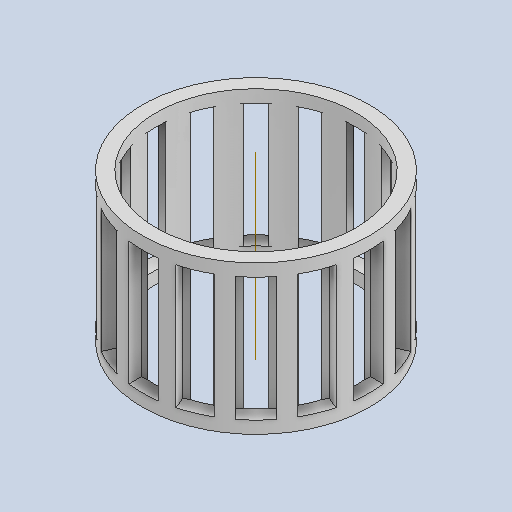
# Autodesk Inventor part: magnet_ring
Saved by Autodesk Inventor 2025 (Build 290162000, 162)
## iProperties
Created: 2026-08-03
Part Number: magnet_ring
Material: Ogólny
Document SubType Name: Modeling
Designer: zzapa
Density: 1 g/cm^3
Appearance: Domyślna
Author: zzapa
Autodesk Inventor part; units mm, degrees
ref_plane "YZ Plane" through (0, 0, 0) normal (1, 0, 0) x (0, 1, 0)
ref_plane "XZ Plane" through (0, 0, 0) normal (0, 1, 0) x (-1, 0, 0)
ref_plane "XY Plane" through (0, 0, 0) normal (0, 0, 1) x (1, 0, 0)
sketch "Szkic1" plane through (0, 0, 0) normal (0, 0, 1) x (1, 0, 0)
  line L0 (27.5, 18) -> (24.2, 18)
  line L1 (24.2, 18) -> (24.2, -18)
  line L2 (24.2, -18) -> (27.5, -18)
  line L3 (27.5, -18) -> (27.5, 18)
  line L4 (-5.5, 0) -> (33, 0) projected
  line L5 (0, -25.2) -> (0, 25.2) projected
  point P0 (0, 0)
  point P1 (24.2, 0)
  dimension "d0" = 27.5
  dimension "d1" = 3.3
  dimension "d15" = 36
  constraints: 8 end point, 2 parallel, 1 horizontal, 1 midpoint, 1 perpendicular, 1 point on line
  measures "d0" distance from line of point (0, 0) L3
  measures "d1" distance of L0.start L0.end
  measures "d15" distance of L2.end L0.start
revolve "Obrót1" add sketch "Szkic1" angle 360 about axis through (0, -10, 0) along (0, 1, 0)
sketch "Szkic2" plane through (0, 0, 0) normal (0, 1, 0) x (-1, 0, 0)
  line L0 (24.1699, -3.55) -> (27.2699, -3.55)
  line L1 (27.2699, -3.55) -> (27.2699, 3.55)
  line L2 (27.2699, 3.55) -> (24.1699, 3.55)
  line L3 (24.1699, 3.55) -> (24.1699, -3.55)
  circle A0 centre (0, 0) radius 27.5 projected
  line L4 (38.5, 0) -> (-38.5, 0) projected
  line L5 (27.2699, -3.55) -> (27.5, -3.55)
  line L6 (27.5, -3.55) -> (27.5, 3.55)
  line L7 (27.5, 3.55) -> (27.2699, 3.55)
  line L8 (27.2699, 3.55) -> (27.2699, -3.55)
  line L9 (24.1043, -2.15) -> (24.1699, -2.15)
  line L10 (24.1699, -2.15) -> (24.1699, 2.15)
  line L11 (24.1699, 2.15) -> (24.1043, 2.15)
  line L12 (24.1043, 2.15) -> (24.1043, -2.15)
  circle A1 centre (0, 0) radius 24.2 projected
  line L13 (23.0922, 7.238) -> (23.1528, 7.2631)
  line L14 (21.4467, 11.2107) -> (23.0922, 7.238)
  line L15 (23.1528, 7.2631) -> (21.5073, 11.2358)
  line L16 (20.9716, 12.5292) -> (23.6886, 5.9696)
  line L17 (23.6886, 5.9696) -> (26.5526, 7.156)
  line L18 (23.8356, 13.7155) -> (20.9716, 12.5292)
  line L19 (26.5526, 7.156) -> (26.7652, 7.244)
  line L20 (24.0482, 13.8036) -> (23.8356, 13.7155)
  line L21 (26.5526, 7.156) -> (23.8356, 13.7155)
  line L22 (23.8356, 13.7155) -> (26.5526, 7.156)
  line L23 (26.7652, 7.244) -> (24.0482, 13.8036)
  line L24 (21.5073, 11.2358) -> (21.4467, 11.2107)
  line L25 (18.5646, 15.524) -> (18.611, 15.5704)
  line L26 (15.524, 18.5646) -> (18.5646, 15.524)
  line L27 (18.611, 15.5704) -> (15.5704, 18.611)
  line L28 (14.5805, 19.6009) -> (19.6009, 14.5805)
  line L29 (19.6009, 14.5805) -> (21.793, 16.7725)
  line L30 (16.7725, 21.793) -> (14.5805, 19.6009)
  line L31 (21.793, 16.7725) -> (21.9557, 16.9352)
  line L32 (16.9352, 21.9557) -> (16.7725, 21.793)
  line L33 (21.793, 16.7725) -> (16.7725, 21.793)
  line L34 (16.7725, 21.793) -> (21.793, 16.7725)
  line L35 (21.9557, 16.9352) -> (16.9352, 21.9557)
  line L36 (15.5704, 18.611) -> (15.524, 18.5646)
  line L37 (11.2107, 21.4467) -> (11.2358, 21.5073)
  line L38 (7.238, 23.0922) -> (11.2107, 21.4467)
  line L39 (11.2358, 21.5073) -> (7.2631, 23.1528)
  line L40 (5.9696, 23.6886) -> (12.5292, 20.9716)
  line L41 (12.5292, 20.9716) -> (13.7155, 23.8356)
  line L42 (7.156, 26.5526) -> (5.9696, 23.6886)
  line L43 (13.7155, 23.8356) -> (13.8036, 24.0482)
  line L44 (7.244, 26.7652) -> (7.156, 26.5526)
  line L45 (13.7155, 23.8356) -> (7.156, 26.5526)
  line L46 (7.156, 26.5526) -> (13.7155, 23.8356)
  line L47 (13.8036, 24.0482) -> (7.244, 26.7652)
  line L48 (7.2631, 23.1528) -> (7.238, 23.0922)
  line L49 (2.15, 24.1043) -> (2.15, 24.1699)
  line L50 (-2.15, 24.1043) -> (2.15, 24.1043)
  line L51 (2.15, 24.1699) -> (-2.15, 24.1699)
  line L52 (-3.55, 24.1699) -> (3.55, 24.1699)
  line L53 (3.55, 24.1699) -> (3.55, 27.2699)
  line L54 (-3.55, 27.2699) -> (-3.55, 24.1699)
  line L55 (3.55, 27.2699) -> (3.55, 27.5)
  line L56 (-3.55, 27.5) -> (-3.55, 27.2699)
  line L57 (3.55, 27.2699) -> (-3.55, 27.2699)
  line L58 (-3.55, 27.2699) -> (3.55, 27.2699)
  line L59 (3.55, 27.5) -> (-3.55, 27.5)
  line L60 (-2.15, 24.1699) -> (-2.15, 24.1043)
  line L61 (-7.238, 23.0922) -> (-7.2631, 23.1528)
  line L62 (-11.2107, 21.4467) -> (-7.238, 23.0922)
  line L63 (-7.2631, 23.1528) -> (-11.2358, 21.5073)
  line L64 (-12.5292, 20.9716) -> (-5.9696, 23.6886)
  line L65 (-5.9696, 23.6886) -> (-7.156, 26.5526)
  line L66 (-13.7155, 23.8356) -> (-12.5292, 20.9716)
  line L67 (-7.156, 26.5526) -> (-7.244, 26.7652)
  line L68 (-13.8036, 24.0482) -> (-13.7155, 23.8356)
  line L69 (-7.156, 26.5526) -> (-13.7155, 23.8356)
  line L70 (-13.7155, 23.8356) -> (-7.156, 26.5526)
  line L71 (-7.244, 26.7652) -> (-13.8036, 24.0482)
  line L72 (-11.2358, 21.5073) -> (-11.2107, 21.4467)
  line L73 (-15.524, 18.5646) -> (-15.5704, 18.611)
  line L74 (-18.5646, 15.524) -> (-15.524, 18.5646)
  line L75 (-15.5704, 18.611) -> (-18.611, 15.5704)
  line L76 (-19.6009, 14.5805) -> (-14.5805, 19.6009)
  line L77 (-14.5805, 19.6009) -> (-16.7725, 21.793)
  line L78 (-21.793, 16.7725) -> (-19.6009, 14.5805)
  line L79 (-16.7725, 21.793) -> (-16.9352, 21.9557)
  line L80 (-21.9557, 16.9352) -> (-21.793, 16.7725)
  line L81 (-16.7725, 21.793) -> (-21.793, 16.7725)
  line L82 (-21.793, 16.7725) -> (-16.7725, 21.793)
  line L83 (-16.9352, 21.9557) -> (-21.9557, 16.9352)
  line L84 (-18.611, 15.5704) -> (-18.5646, 15.524)
  line L85 (-21.4467, 11.2107) -> (-21.5073, 11.2358)
  line L86 (-23.0922, 7.238) -> (-21.4467, 11.2107)
  line L87 (-21.5073, 11.2358) -> (-23.1528, 7.2631)
  line L88 (-23.6886, 5.9696) -> (-20.9716, 12.5292)
  line L89 (-20.9716, 12.5292) -> (-23.8356, 13.7155)
  line L90 (-26.5526, 7.156) -> (-23.6886, 5.9696)
  line L91 (-23.8356, 13.7155) -> (-24.0482, 13.8036)
  line L92 (-26.7652, 7.244) -> (-26.5526, 7.156)
  line L93 (-23.8356, 13.7155) -> (-26.5526, 7.156)
  line L94 (-26.5526, 7.156) -> (-23.8356, 13.7155)
  line L95 (-24.0482, 13.8036) -> (-26.7652, 7.244)
  line L96 (-23.1528, 7.2631) -> (-23.0922, 7.238)
  line L97 (-24.1043, 2.15) -> (-24.1699, 2.15)
  line L98 (-24.1043, -2.15) -> (-24.1043, 2.15)
  line L99 (-24.1699, 2.15) -> (-24.1699, -2.15)
  line L100 (-24.1699, -3.55) -> (-24.1699, 3.55)
  line L101 (-24.1699, 3.55) -> (-27.2699, 3.55)
  line L102 (-27.2699, -3.55) -> (-24.1699, -3.55)
  line L103 (-27.2699, 3.55) -> (-27.5, 3.55)
  line L104 (-27.5, -3.55) -> (-27.2699, -3.55)
  line L105 (-27.2699, 3.55) -> (-27.2699, -3.55)
  line L106 (-27.2699, -3.55) -> (-27.2699, 3.55)
  line L107 (-27.5, 3.55) -> (-27.5, -3.55)
  line L108 (-24.1699, -2.15) -> (-24.1043, -2.15)
  line L109 (-23.0922, -7.238) -> (-23.1528, -7.2631)
  line L110 (-21.4467, -11.2107) -> (-23.0922, -7.238)
  line L111 (-23.1528, -7.2631) -> (-21.5073, -11.2358)
  line L112 (-20.9716, -12.5292) -> (-23.6886, -5.9696)
  line L113 (-23.6886, -5.9696) -> (-26.5526, -7.156)
  line L114 (-23.8356, -13.7155) -> (-20.9716, -12.5292)
  line L115 (-26.5526, -7.156) -> (-26.7652, -7.244)
  line L116 (-24.0482, -13.8036) -> (-23.8356, -13.7155)
  line L117 (-26.5526, -7.156) -> (-23.8356, -13.7155)
  line L118 (-23.8356, -13.7155) -> (-26.5526, -7.156)
  line L119 (-26.7652, -7.244) -> (-24.0482, -13.8036)
  line L120 (-21.5073, -11.2358) -> (-21.4467, -11.2107)
  line L121 (-18.5646, -15.524) -> (-18.611, -15.5704)
  line L122 (-15.524, -18.5646) -> (-18.5646, -15.524)
  line L123 (-18.611, -15.5704) -> (-15.5704, -18.611)
  line L124 (-14.5805, -19.6009) -> (-19.6009, -14.5805)
  line L125 (-19.6009, -14.5805) -> (-21.793, -16.7725)
  line L126 (-16.7725, -21.793) -> (-14.5805, -19.6009)
  line L127 (-21.793, -16.7725) -> (-21.9557, -16.9352)
  line L128 (-16.9352, -21.9557) -> (-16.7725, -21.793)
  line L129 (-21.793, -16.7725) -> (-16.7725, -21.793)
  line L130 (-16.7725, -21.793) -> (-21.793, -16.7725)
  line L131 (-21.9557, -16.9352) -> (-16.9352, -21.9557)
  line L132 (-15.5704, -18.611) -> (-15.524, -18.5646)
  line L133 (-11.2107, -21.4467) -> (-11.2358, -21.5073)
  line L134 (-7.238, -23.0922) -> (-11.2107, -21.4467)
  line L135 (-11.2358, -21.5073) -> (-7.2631, -23.1528)
  line L136 (-5.9696, -23.6886) -> (-12.5292, -20.9716)
  line L137 (-12.5292, -20.9716) -> (-13.7155, -23.8356)
  line L138 (-7.156, -26.5526) -> (-5.9696, -23.6886)
  line L139 (-13.7155, -23.8356) -> (-13.8036, -24.0482)
  line L140 (-7.244, -26.7652) -> (-7.156, -26.5526)
  line L141 (-13.7155, -23.8356) -> (-7.156, -26.5526)
  line L142 (-7.156, -26.5526) -> (-13.7155, -23.8356)
  line L143 (-13.8036, -24.0482) -> (-7.244, -26.7652)
  line L144 (-7.2631, -23.1528) -> (-7.238, -23.0922)
  line L145 (-2.15, -24.1043) -> (-2.15, -24.1699)
  line L146 (2.15, -24.1043) -> (-2.15, -24.1043)
  line L147 (-2.15, -24.1699) -> (2.15, -24.1699)
  line L148 (3.55, -24.1699) -> (-3.55, -24.1699)
  line L149 (-3.55, -24.1699) -> (-3.55, -27.2699)
  line L150 (3.55, -27.2699) -> (3.55, -24.1699)
  line L151 (-3.55, -27.2699) -> (-3.55, -27.5)
  line L152 (3.55, -27.5) -> (3.55, -27.2699)
  line L153 (-3.55, -27.2699) -> (3.55, -27.2699)
  line L154 (3.55, -27.2699) -> (-3.55, -27.2699)
  line L155 (-3.55, -27.5) -> (3.55, -27.5)
  line L156 (2.15, -24.1699) -> (2.15, -24.1043)
  line L157 (7.238, -23.0922) -> (7.2631, -23.1528)
  line L158 (11.2107, -21.4467) -> (7.238, -23.0922)
  line L159 (7.2631, -23.1528) -> (11.2358, -21.5073)
  line L160 (12.5292, -20.9716) -> (5.9696, -23.6886)
  line L161 (5.9696, -23.6886) -> (7.156, -26.5526)
  line L162 (13.7155, -23.8356) -> (12.5292, -20.9716)
  line L163 (7.156, -26.5526) -> (7.244, -26.7652)
  line L164 (13.8036, -24.0482) -> (13.7155, -23.8356)
  line L165 (7.156, -26.5526) -> (13.7155, -23.8356)
  line L166 (13.7155, -23.8356) -> (7.156, -26.5526)
  line L167 (7.244, -26.7652) -> (13.8036, -24.0482)
  line L168 (11.2358, -21.5073) -> (11.2107, -21.4467)
  line L169 (15.524, -18.5646) -> (15.5704, -18.611)
  line L170 (18.5646, -15.524) -> (15.524, -18.5646)
  line L171 (15.5704, -18.611) -> (18.611, -15.5704)
  line L172 (19.6009, -14.5805) -> (14.5805, -19.6009)
  line L173 (14.5805, -19.6009) -> (16.7725, -21.793)
  line L174 (21.793, -16.7725) -> (19.6009, -14.5805)
  line L175 (16.7725, -21.793) -> (16.9352, -21.9557)
  line L176 (21.9557, -16.9352) -> (21.793, -16.7725)
  line L177 (16.7725, -21.793) -> (21.793, -16.7725)
  line L178 (21.793, -16.7725) -> (16.7725, -21.793)
  line L179 (16.9352, -21.9557) -> (21.9557, -16.9352)
  line L180 (18.611, -15.5704) -> (18.5646, -15.524)
  line L181 (21.4467, -11.2107) -> (21.5073, -11.2358)
  line L182 (23.0922, -7.238) -> (21.4467, -11.2107)
  line L183 (21.5073, -11.2358) -> (23.1528, -7.2631)
  line L184 (23.6886, -5.9696) -> (20.9716, -12.5292)
  line L185 (20.9716, -12.5292) -> (23.8356, -13.7155)
  line L186 (26.5526, -7.156) -> (23.6886, -5.9696)
  line L187 (23.8356, -13.7155) -> (24.0482, -13.8036)
  line L188 (26.7652, -7.244) -> (26.5526, -7.156)
  line L189 (23.8356, -13.7155) -> (26.5526, -7.156)
  line L190 (26.5526, -7.156) -> (23.8356, -13.7155)
  line L191 (24.0482, -13.8036) -> (26.7652, -7.244)
  line L192 (23.1528, -7.2631) -> (23.0922, -7.238)
  point P0 (27.2699, 0)
  point P1 (27.5, 0)
  point P2 (24.1043, 0)
  point P3 (22.2695, 9.2243)
  point P4 (25.1941, 10.4357)
  point P5 (25.4067, 10.5238)
  point P6 (17.0443, 17.0443)
  point P7 (19.2827, 19.2827)
  point P8 (19.4454, 19.4454)
  point P9 (9.2243, 22.2695)
  point P10 (10.4357, 25.1941)
  point P11 (10.5238, 25.4067)
  point P12 (0, 24.1043)
  point P13 (0, 27.2699)
  point P14 (0, 27.5)
  point P15 (-9.2243, 22.2695)
  point P16 (-10.4357, 25.1941)
  point P17 (-10.5238, 25.4067)
  point P18 (-17.0443, 17.0443)
  point P19 (-19.2827, 19.2827)
  point P20 (-19.4454, 19.4454)
  point P21 (-22.2695, 9.2243)
  point P22 (-25.1941, 10.4357)
  point P23 (-25.4067, 10.5238)
  point P24 (-24.1043, 0)
  point P25 (-27.2699, 0)
  point P26 (-27.5, 0)
  point P27 (-22.2695, -9.2243)
  point P28 (-25.1941, -10.4357)
  point P29 (-25.4067, -10.5238)
  point P30 (-17.0443, -17.0443)
  point P31 (-19.2827, -19.2827)
  point P32 (-19.4454, -19.4454)
  point P33 (-9.2243, -22.2695)
  point P34 (-10.4357, -25.1941)
  point P35 (-10.5238, -25.4067)
  point P36 (0, -24.1043)
  point P37 (0, -27.2699)
  point P38 (0, -27.5)
  point P39 (9.2243, -22.2695)
  point P40 (10.4357, -25.1941)
  point P41 (10.5238, -25.4067)
  point P42 (17.0443, -17.0443)
  point P43 (19.2827, -19.2827)
  point P44 (19.4454, -19.4454)
  point P45 (22.2695, -9.2243)
  point P46 (25.1941, -10.4357)
  point P47 (25.4067, -10.5238)
  dimension "d3" = 7.1
  dimension "d4" = 3.1
  dimension "d16" = 1.4
  dimension "d19" = 360
  constraints: 384 end point, 6 parallel, 3 horizontal, 3 midpoint, 3 perpendicular, 2 collinear, 2 point on circle, 2 point on line, 419 other
  measures "d3" distance of L0.end L1.end
  measures "d4" distance of L1.end L2.end
  measures "d16" distance between parallel lines of L11 L2
extrude "Pocket" cut sketch "Szkic2" along normal mid plane 30 contours L3 A1 L4 L1 L0 | L1 L4 A0 | A0 L6 L5 | L9 A1 L3 | L4 A1 L3 L2 L1 | L1 A0 L4 | L188 L191 A0 | L189 L185 L184 L183 A1 L186 | A0 L189 | A0 L7 L6 | A1 L12 L4 L3 | L3 L4 A1 | A1 L182 L170 L158 L146 L134 L122 L110 L98 L4 L12 | L4 L3 A1 | L191 L187 A0 | L4 L12 A1 L3 | L4 L98 A1 L86 L74 L62 L50 L38 L26 L14 L12 | L192 L183 A1 | A1 L183 L182 | L21 A0 | A0 L23 L19 | L17 L16 L15 A1 L18 L21 | A1 L11 L3 | L176 L179 A0 | L177 L173 L172 L171 A1 L174 | A0 L177 | L98 A1 L99 L4 | L4 L99 A1 L98 | A1 L183 | A1 L183 L181 | A0 L20 L23 | L179 L175 A0 | L99 A1 L4 | L4 A1 L99 | L108 L99 A1 | A1 L99 L97 | L14 A1 L15 | A1 L15 L13 | L180 L171 A1 | A1 L171 L170 | L33 A0 | A0 L35 L31 | L29 L28 L27 A1 L30 L33 | L164 L167 A0 | L165 L161 L160 L159 A1 L162 | A0 L165 | A1 L99 L100 L102 A0 L4 | L4 A0 L101 L100 L99 A1 | L110 A1 L111 | A1 L111 L109 | L96 L87 A1 | A1 L87 L86 | L15 A1 | L24 L15 A1 | A1 L171 | A1 L171 L169 | A0 L32 L35 | L167 L163 A0 | L111 A1 | A1 L111 L112 L114 L117 L113 | L120 L111 A1 | L87 L88 L90 L93 L89 A1 | A1 L87 | A1 L87 L85 | L26 A1 L27 | A1 L27 L25 | L168 L159 A1 | A1 L159 L158 | L45 A0 | A0 L47 L43 | L41 L40 L39 A1 L42 L45 | L152 L155 A0 | L153 L149 L148 L147 A1 L150 | A0 L153 | L122 A1 L123 | A1 L123 L121 | L84 L75 A1 | A1 L75 L74 | L27 A1 | L36 L27 A1 | A1 L159 | A1 L159 L157 | A0 L44 L47 | L155 L151 A0 | L92 L95 A0 | A0 L93 | L117 A0 | A0 L119 L115 | L123 A1 | A1 L123 L124 L126 L129 L125 | L132 L123 A1 | L75 L76 L78 L81 L77 A1 | A1 L75 | A1 L75 L73 | L38 A1 L39 | A1 L39 L37 | L156 L147 A1 | A1 L147 L146 | L57 A0 | A0 L59 L55 | L53 L52 L51 A1 L54 L57 | L140 L143 A0 | L141 L137 L136 L135 A1 L138 | A0 L141 | L95 L91 A0 | A0 L116 L119 | L134 A1 L135 | A1 L135 L133 | L72 L63 A1 | A1 L63 L62 | L39 A1 | L48 L39 A1 | A1 L147 | A1 L147 L145 | A0 L56 L59 | L143 L139 A0 | L80 L83 A0 | A0 L81 | L129 A0 | A0 L131 L127 | L135 A1 | L144 L135 A1 | L63 L64 L66 L69 L65 A1 | A1 L63 | A1 L63 L61 | L50 A1 L51 | A1 L51 L49 | L69 A0 | A0 L71 L67 | L128 L131 A0 | L83 L79 A0 | L60 L51 A1 | L51 A1 | A0 L68 L71
equation "\"d0\" = magnet_ring_r"
equation "\"d1\" = magnet_ring_d"
equation "\"d15\" = magnet_ring_h"
equation "\"d3\" = magnet_ring_pocket_mag_size_x"
equation "\"d4\" = magnet_ring_pocket_mag_size_y"
equation "\"d16\" = magnet_ring_pocket_radial_cut"
equation "\"stator_out_d\" = 2.5"
equation "\"stator_h\" = 35"
equation "\"mag_size_x\" = 7"
equation "\"mag_size_y\" = 3"
equation "\"mag_corner_r\" = 0.4"
equation "\"magnet_ring_r\" = 27.5"
equation "\"magnet_ring_d\" = 3.3"
equation "\"magnet_ring_pocket_mag_size_y\" = 3.1"
equation "\"magnet_ring_pocket_mag_size_x\" = 7.1"
equation "\"magnet_ring_pocket_mag_size_z\" = 10.3"
equation "\"magnet_ring_mag_count\" = 16"
equation "\"magnet_ring_h\" = 36"
equation "\"magnet_ring_pocket_radial_cut\" = 1.4"
equation "\"casing_d\" = 3"
equation "\"rotor_core_r\" = 15"
equation "\"coil_groove_ang\" = 18"
equation "\"rotor_out_r\" = 23"
equation "\"rotor_coil_groove_in_r\" = 17"
equation "\"rotor_coil_groove_ang\" = 18deg"
equation "\"rotor_coil_groove_in_correction_r\" = 18"
equation "\"rotor_plastic_h\" = 32"
equation "\"rotor_teeth_d\" = 1.5"
equation "\"shaft_d\" = 8"
equation "\"insert25m_d\" = 2.9"
equation "\"insert25m_corner\" = 0.5"
equation "\"insert25m_h\" = 7"
equation "\"rotor_plastic_insert_r\" = 37"
equation "\"shaft_lock_1_d\" = 8"
equation "\"shaf_lock_1_D\" = 32"
equation "\"shaft_lock_1_D\" = 36"
equation "\"shaft_lock_1_h1\" = 4"
equation "\"shaft_lock_1_insert_part_h\" = 7"
equation "\"shaft_lock_1_corner\" = 1"
equation "\"shaft_lock_1_insert_part_a\" = 18"
equation "\"shaft_lock_2_h1\" = 4"
equation "\"shaft_lock_2_d\" = 7"
equation "\"shaft_lock_2_insert_part_a\" = 18"
equation "\"shaft_lock_2_D\" = 44"
equation "\"shaft_lock_2_corner\" = 1"
equation "\"shaft_lock_2_insert_part_h\" = 7"
equation "\"shaft_lock_2_rotor_insert_grove_d_in\" = 36"
equation "\"shaft_lock_2_rotor_insert_grove_width_out\" = 5.5"
equation "\"shaft_lock_2_rotor_insert_grove_width_in\" = 7.6"
equation "\"shaft_lock_2_rotor_insert_r\" = 37"
equation "\"shaft_lock_2_rotor_insert_screw_d\" = 2.6"
equation "\"insert25m_pocket_d\" = 2.6"
equation "\"insert25m_pocket_D\" = 4.5"
equation "\"insert25m_pocket_nut_h\" = 1.5"
equation "\"insert_m2_pocket_d\" = 2.6"
equation "\"insert_m2_h\" = 7"
equation "\"insert_m2_d\" = 2.9"
equation "\"insert_m2_corner\" = 0.5"
equation "\"insert_m2_pocket_D\" = 4.5"
equation "\"insert_m2_pocket_nut_h\" = 1.5"
